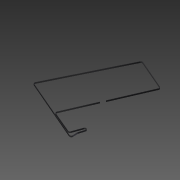
# Autodesk Inventor part: BeltRight
Saved by Autodesk Inventor 2015 (Build 190159000, 159)
## iProperties
Created: 2014-08-13
Part Number: BeltRight
Material: Rubber
Document SubType Name: Modeling
Designer: t_clevj
Density: 0.93 g/cm^3
Appearance: Rubber - Black - Version 1.1
Author: t_clevj
Autodesk Inventor part; units mm, degrees
ref_plane "YZ Plane" through (0, 0, 0) normal (1, 0, 0) x (0, 1, 0)
ref_plane "XZ Plane" through (0, 0, 0) normal (0, 1, 0) x (-1, 0, 0)
ref_plane "XY Plane" through (0, 0, 0) normal (0, 0, 1) x (1, 0, 0)
sketch "Sketch1" plane through (0, 0, 0) normal (0, 0, 1) x (1, 0, 0)
  circle A0 centre (0, 0) radius 7.5 projected
  circle A1 centre (4.7555, -31.9787) radius 6.5 projected
  circle A2 centre (-29.46, -40.6707) radius 6.5 projected
  circle A3 centre (-8.4678, -55.1389) radius 6.5 projected
  circle A4 centre (-67.1261, -24.4762) radius 7.4 projected
  circle A5 centre (-305.2033, 72.4426) radius 6.5 projected
  circle A6 centre (-140.546, 409.84) radius 6.5 projected
  circle A7 centre (65.2396, 321.3624) radius 6.5 projected
  circle A8 centre (0, 0) radius 6 construction
  line L0 (5.7316, -1.7744) -> (-2.8867, -29.6128)
  arc A9 (-2.8867, -29.6128) -> (-3.232, -32.4269) centre (4.7555, -31.9787) ccw
  line L1 (-3.232, -32.4269) -> (-1.978, -54.7747)
  line L2 (-11.0352, -61.1103) -> (-307.7707, 66.4712)
  line L3 (-311.0448, 75.2934) -> (-146.3875, 412.6908)
  line L4 (-137.9786, 415.8114) -> (67.807, 327.3339)
  line L5 (71.2111, 318.795) -> (15.5452, 189.3244)
  line L6 (-5.6477, 2.0256) -> (-21.9297, -43.3715)
  arc A10 (-32.4578, -48.0878) -> (-21.9297, -43.3715) centre (-29.46, -40.6707) ccw
  line L7 (-32.4578, -48.0878) -> (-70.4612, -32.7277)
  arc A11 (-75.3024, -20.9608) -> (-70.4612, -32.7277) centre (-67.1261, -24.4762) ccw
  line L8 (-75.3024, -20.9608) -> (8.905, 174.893)
  arc A12 (-311.0448, 75.2934) -> (-307.7707, 66.4712) centre (-305.2033, 72.4426) ccw
  arc A13 (-137.9786, 415.8114) -> (-146.3875, 412.6908) centre (-140.546, 409.84) ccw
  arc A14 (71.2111, 318.795) -> (67.807, 327.3339) centre (65.2396, 321.3624) ccw
  arc A15 (5.7316, -1.7744) -> (-5.6477, 2.0256) centre (0, 0) ccw
  arc A16 (-11.0352, -61.1103) -> (-1.978, -54.7747) centre (-8.4678, -55.1389) ccw
  line L9 (16.9232, 188.7319) -> (72.5891, 318.2025)
  arc A17 (72.5891, 318.2025) -> (68.3995, 328.7119) centre (65.2396, 321.3624) ccw
  line L10 (68.3995, 328.7119) -> (-137.3861, 417.1895)
  arc A18 (-137.3861, 417.1895) -> (-147.7355, 413.3486) centre (-140.546, 409.84) ccw
  line L11 (-147.7355, 413.3486) -> (-312.3928, 75.9513)
  arc A19 (-312.3928, 75.9513) -> (-308.3632, 65.0932) centre (-305.2033, 72.4426) ccw
  line L12 (-308.3632, 65.0932) -> (-11.6277, -62.4884)
  arc A20 (-11.6277, -62.4884) -> (-0.4804, -54.6907) centre (-8.4678, -55.1389) ccw
  line L13 (-0.4804, -54.6907) -> (-1.7343, -32.3428)
  arc A21 (-1.4538, -30.0564) -> (-1.7343, -32.3428) centre (4.7555, -31.9787) ccw
  line L14 (-1.4538, -30.0564) -> (7.1645, -2.218)
  arc A22 (7.1645, -2.218) -> (-7.0597, 2.532) centre (0, 0) ccw
  line L15 (-7.0597, 2.532) -> (-23.3416, -42.8651)
  arc A23 (-31.8957, -46.6971) -> (-23.3416, -42.8651) centre (-29.46, -40.6707) ccw
  line L16 (-31.8957, -46.6971) -> (-69.8991, -31.337)
  arc A24 (-73.9244, -21.5533) -> (-69.8991, -31.337) centre (-67.1261, -24.4762) ccw
  line L17 (-73.9244, -21.5533) -> (10.283, 174.3005)
  line L18 (8.905, 174.893) -> (10.283, 174.3005)
  line L19 (15.5452, 189.3244) -> (16.9232, 188.7319)
  point P0 (0, 0)
  dimension "d0" = 12
  dimension "d1" = 1.5
  dimension "d2" = 1.5
  dimension "d3" = 1.5
  dimension "d4" = 1.5
  constraints: 42 point on circle, 40 end point, 22 tangent, 17 centre point, 5 perpendicular, 4 coincident, 3 concentric, 1 parallel, 16 other
  measures "d0" diameter of A8
  measures "d1" radial gap between concentric circles of A2 A10
  measures "d2" radial gap between concentric circles of A4 A11
  measures "d3" radial gap between concentric circles of A1 A9
  measures "d4" distance between parallel lines of L1 L13
extrude "Extrusion1" add sketch "Sketch1" along normal blind 6 contours A0 L0 A15 L6 | A0 L6 A10 L7 A11 L8 L18 L17 A4 L16 A2 L15 | L14 A1 L13 A20 L12 A19 L11 A18 L10 A17 L9 L19 L5 A7 L4 A6 L3 A5 L2 A3 L1 A9 L0 A0 picked at (-6.7626, -0.2729)
body "Solid1"
